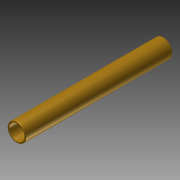
# Autodesk Inventor part: Rudder_Hinge_Pipe
Saved by Autodesk Inventor 2011 SP1 (Build 150282100, 282)
## iProperties
Created: 2011-06-11
Part Number: Rudder_Hinge_Pipe
Document SubType Name: Modeling
Designer: Andrew G. Meyer
Mass: 0.211091 g
Surface Area: 10.4788 cm^2
Volume: 0.211091 cm^3
Density: 1 g/cm^3
Author: Andrew G. Meyer
Autodesk Inventor part; units mm, degrees
ref_plane "YZ Plane" through (0, 0, 0) normal (1, 0, 0) x (0, 1, 0)
ref_plane "XZ Plane" through (0, 0, 0) normal (0, 1, 0) x (-1, 0, 0)
ref_plane "XY Plane" through (0, 0, 0) normal (0, 0, 1) x (1, 0, 0)
sketch "Sketch1" plane through (0, 0, 0) normal (0, 0, 1) x (1, 0, 0)
  circle A0 centre (0, 0) radius 2.3749
  circle A1 centre (0, 0) radius 1.9685
  dimension "d0" = 4.7498
  dimension "d1" = 0.4064
  constraints: 2 centre point, 2 coincident
  measures "d0" diameter of A0
  measures "d1" radial gap between concentric circles of A0 A1
extrude "Extrusion1" add sketch "Sketch1" along normal blind 38.1
fillet "Fillet1" radius 0.127 4 edges at (-2.3749, 0, 38.1) (-1.9685, 0, 38.1) (-1.9685, 0, 0) (-2.3749, 0, 0)
body "Solid1"
